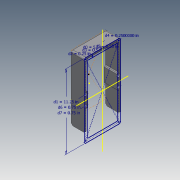
# Autodesk Inventor part: Standard
Saved by Autodesk Inventor 2020.3 (Build 243373000, 373)
## iProperties
RuleStatus: InUse
AfterDocSave0: file://Part Number Cleaner
Created: 2023-01-17
Material: Generic
Catalog Web Link: https://www.janelia.org/
Vendor: HHMI: JRC - jET
Document SubType Name: Modeling
Designer: arnoldj
Density: 1 g/cm^3
Appearance: Default
LAB/DEPT: A. LEE (LAB)
DESIGN DEPARTMENT: HHMI: JRC - jET
ALTERED ITEM PART NUMBER: N/A
ALTERED ITEM VENDOR: N/A
ALTERED ITEM DESCRIPTION: N/A
Title: Standard
Author: arnoldj
Revision Number: 0
Autodesk Inventor part; units mm, degrees
ref_plane "YZ Plane" through (0, 0, 0) normal (1, 0, 0) x (0, 1, 0)
ref_plane "XZ Plane" through (0, 0, 0) normal (0, 1, 0) x (-1, 0, 0)
ref_plane "XY Plane" through (0, 0, 0) normal (0, 0, 1) x (1, 0, 0)
sketch "Sketch1" plane through (0, 0, 0) normal (1, 0, 0) x (0, 1, 0)
  line L0 (0, 99.6312) -> (0, -99.6312) projected
  line L1 (-202.2597, 0) -> (204.2274, 0) projected
  line L2 (-136.525, -69.85) -> (136.525, -69.85)
  line L3 (142.875, -63.5) -> (142.875, 63.5)
  line L4 (136.525, 69.85) -> (-136.525, 69.85)
  line L5 (-142.875, 63.5) -> (-142.875, -63.5)
  line L6 (-142.875, -69.85) -> (142.875, 69.85) construction
  line L7 (142.875, -69.85) -> (-142.875, 69.85) construction
  arc A0 (142.875, 63.5) -> (136.525, 69.85) centre (136.525, 63.5) ccw
  arc A1 (136.525, -69.85) -> (142.875, -63.5) centre (136.525, -63.5) ccw
  arc A2 (-142.875, -63.5) -> (-136.525, -69.85) centre (-136.525, -63.5) ccw
  arc A3 (-136.525, 69.85) -> (-142.875, 63.5) centre (-136.525, 63.5) ccw
  line L8 (130.175, 57.15) -> (130.175, -57.15)
  line L9 (130.175, -57.15) -> (-130.175, -57.15)
  line L10 (-130.175, -57.15) -> (-130.175, 57.15)
  line L11 (-130.175, 57.15) -> (130.175, 57.15)
  line L12 (-136.525, 63.5) -> (136.525, 63.5) construction
  line L13 (136.525, 63.5) -> (136.525, -63.5) construction
  line L14 (136.525, -63.5) -> (-136.525, -63.5) construction
  line L15 (-136.525, -63.5) -> (-136.525, 63.5) construction
  line L16 (-136.525, 63.5) -> (136.525, -63.5) construction
  line L17 (136.525, 63.5) -> (-136.525, -63.5) construction
  point P0 (0, 0)
  point P1 (19.05, 63.5)
  point P2 (19.05, -63.5)
  point P3 (-19.05, 63.5)
  point P4 (-19.05, -63.5)
  dimension "d0" = 139.7
  dimension "d1" = 285.75
  dimension "d2" = 6.35
  dimension "d3" = 12.7
  dimension "d4" = 6.35
  dimension "d5" = 6.35
  dimension "d6" = 19.05
  dimension "d7" = 19.05
  constraints: 32 end point, 12 point on line, 8 point on circle, 8 tangent, 6 parallel, 4 centre point, 4 coincident, 4 midpoint, 3 equal radius, 3 perpendicular, 2 horizontal, 2 vertical alignment, 3 other
  measures "d0" distance of L7.start L6.end
  measures "d1" distance of L6.end L7.end
  measures "d2" radius of A0
  measures "d3" distance between parallel lines of L3 L8
  measures "d4" distance between parallel lines of L14 L2
  measures "d5" distance between parallel lines of L13 L3
  measures "d6" distance from line of L0 point (19.05, 63.5)
  measures "d7" distance from line of point (-19.05, 63.5) L0
extrude "Extrusion1" add sketch "Sketch1" against normal blind 49.53 contours L4 A0 L3 L1 L8 L11 L0 | L0 L11 L10 L1 L5 A3 L4 | L9 L8 L1 L3 A1 L2 L0 | L0 L2 A2 L5 L1 L10 L9
fillet "Fillet1" radius 6.35 4 edges at (-24.765, 130.175, 57.15) (-24.765, 130.175, -57.15) (-24.765, -130.175, -57.15) (-24.765, -130.175, 57.15)
hole "Hole1" at (0, 136.525, 63.5) at (0, 136.525, -63.5) at (0, 19.05, 63.5) at (0, 19.05, -63.5) at (0, -19.05, 63.5) at (0, -19.05, -63.5) at (0, -136.525, 63.5) at (0, -136.525, -63.5) direction (-1, 0, 0) diameter 5.334 end through all counterbore diameter 10.16 counterbore depth 8.89
sketch "Sketch2" plane through (-49.53, 0, 0) normal (-1, 0, 0) x (0, 0, 1)
  line L0 (0, -202.2597) -> (0, 204.2274) projected
  line L1 (99.6312, 0) -> (-99.6312, 0) projected
  line L2 (119.4093, -203.1024) -> (-119.4093, -203.1024)
  line L3 (-119.4093, -203.1024) -> (-119.4093, 0)
  line L4 (-119.4093, 0) -> (119.4093, 0)
  line L5 (119.4093, 0) -> (119.4093, -203.1024)
  line L6 (119.4093, -203.1024) -> (-119.4093, 0) construction
  line L7 (-119.4093, -203.1024) -> (119.4093, 0) construction
  point P0 (0, 0)
  point P1 (0, -101.5512)
  point P2 (119.4093, 0)
  dimension "d18" = 0
  constraints: 12 end point, 2 midpoint, 2 parallel, 1 horizontal, 1 perpendicular, 1 point on line
  measures "d18" distance between parallel lines of L4 L1
extrude "Extrusion2" [suppressed]
sketch "Sketch3" plane through (-34.925, 0, -69.85) normal (0, -1, 0) x (1, 0, 0)
  line L0 (0, 12.7) -> (34.925, 12.7) projected
  line L1 (0, 0) -> (0, 12.7) projected
  line L2 (34.925, 0) -> (0, 0) projected
  line L3 (34.925, 12.7) -> (34.925, 0) projected
  line L4 (34.925, 127) -> (0, 127) projected
  line L5 (34.925, 139.7) -> (34.925, 127) projected
  line L6 (0, 139.7) -> (34.925, 139.7) projected
  line L7 (0, 127) -> (0, 139.7) projected
  line L8 (0, 133.35) -> (0, 6.35) construction
  line L9 (34.925, 6.35) -> (0, 6.35) construction
  line L10 (0, 6.35) -> (34.925, 6.35) construction
  line L11 (0, 133.35) -> (34.925, 133.35) construction
  line L12 (34.925, 135.417) -> (34.925, 131.283) construction
  line L13 (34.925, 133.35) -> (0, 133.35) construction
  point P0 (34.925, 69.85)
  point P1 (7.62, 6.35)
  point P2 (27.305, 6.35)
  point P3 (27.305, 133.35)
  point P4 (7.62, 133.35)
  dimension "d21" = 7.62
  dimension "d22" = 7.62
  dimension "d23" = 7.62
  dimension "d24" = 7.62
  constraints: 4 end point, 4 point on line, 1 collinear, 1 midpoint
  measures "d21" distance from line of L1 point (7.62, 6.35)
  measures "d22" distance from line of point (27.305, 6.35) L3
  measures "d23" distance from line of point (7.62, 133.35) L7
  measures "d24" distance from line of point (27.305, 133.35) L5
hole "Hole2" [suppressed]
chamfer "Chamfer1" [suppressed]
sketch "Sketch4" plane through (-49.53, 0, 0) normal (-1, 0, 0) x (0, 0, 1)
  line L0 (0, -202.2597) -> (0, 204.2274) projected
  line L1 (99.6312, 0) -> (-99.6312, 0) projected
  line L2 (116.354, -104.775) -> (-116.354, -104.775)
  line L3 (-116.354, -104.775) -> (-116.354, -199.2224)
  line L4 (-116.354, -199.2224) -> (116.354, -199.2224)
  line L5 (116.354, -199.2224) -> (116.354, -104.775)
  line L6 (116.354, -104.775) -> (-116.354, -199.2224) construction
  line L7 (-116.354, -104.775) -> (116.354, -199.2224) construction
  line L8 (63.5, 142.875) -> (-63.5, 142.875) projected
  point P0 (0, 0)
  point P1 (0, -151.9987)
  dimension "d35" = 247.65
  constraints: 12 end point, 2 midpoint, 2 parallel, 1 horizontal, 1 perpendicular, 1 point on line
  measures "d35" distance between parallel lines of L2 L8
extrude "Extrusion3" cut sketch "Sketch4" against normal through all
sketch "Sketch5" plane through (-49.53, 0, 0) normal (-1, 0, 0) x (0, 0, 1)
  line L0 (-57.15, -104.775) -> (-57.15, 123.825) projected
  line L1 (-50.8, 130.175) -> (50.8, 130.175) projected
  line L2 (57.15, 123.825) -> (57.15, -104.775) projected
  line L3 (0, -202.2597) -> (0, 204.2274) projected
  arc A0 (-50.8, 130.175) -> (-57.15, 123.825) centre (-50.8, 123.825) ccw projected
  arc A1 (57.15, 123.825) -> (50.8, 130.175) centre (50.8, 123.825) ccw projected
  line L4 (-62.23, -104.775) -> (-62.23, 123.825)
  arc A2 (-50.8, 135.255) -> (-62.23, 123.825) centre (-50.8, 123.825) ccw
  line L5 (-50.8, 135.255) -> (50.8, 135.255)
  arc A3 (62.23, 123.825) -> (50.8, 135.255) centre (50.8, 123.825) ccw
  line L6 (62.23, 123.825) -> (62.23, -104.775)
  line L7 (62.23, -28.575) -> (-62.23, -28.575)
  line L8 (-62.23, -28.575) -> (-62.23, 28.575)
  line L9 (-62.23, 28.575) -> (62.23, 28.575)
  line L10 (62.23, 28.575) -> (62.23, -28.575)
  line L11 (62.23, -28.575) -> (-62.23, 28.575) construction
  line L12 (-62.23, -28.575) -> (62.23, 28.575) construction
  line L13 (-69.85, -104.775) -> (-57.15, -104.775) projected
  line L14 (57.15, -104.775) -> (69.85, -104.775) projected
  point P0 (0, 0)
  point P1 (57.15, 28.575)
  point P2 (-57.15, 28.575)
  point P3 (57.15, -28.575)
  point P4 (-57.15, -28.575)
  dimension "d38" = 5.08
  dimension "d39" = 57.15
  constraints: 18 end point, 4 point on circle, 2 centre point, 2 midpoint, 2 parallel, 1 horizontal, 1 perpendicular, 1 point on line, 4 other
  measures "d38" distance between parallel lines of L1 L5
  measures "d39" distance between parallel lines of L7 L9
extrude "Extrusion4" cut sketch "Sketch5" against normal through all contours L13 L4 L7 L0 | L9 L4 A2 L5 L3 L1 A0 L0 | L7 L6 L14 L2 | L3 L5 A3 L6 L9 L2 A1 L1
fillet "Fillet2" radius 3.175 8 edges at (-24.765, -28.575, -57.15) (-24.765, -28.575, -62.23) (-24.765, 28.575, -57.15) (-24.765, 28.575, -62.23) (-24.765, -28.575, 57.15) (-24.765, -28.575, 62.23) (-24.765, 28.575, 57.15) (-24.765, 28.575, 62.23)
chamfer "Chamfer2" distance 6.35 angle 45 2 edges at (-49.53, -104.775, -66.04) (-49.53, -104.775, 66.04)
sketch "Sketch6" plane through (-49.53, 0, 0) normal (-1, 0, 0) x (0, 0, 1)
  line L0 (69.0599, 146.1578) -> (-63.5, 146.1578) construction
  line L1 (-63.5, 146.1578) -> (-63.5, -84.3884) construction
  line L2 (-63.5, -84.3884) -> (69.0599, -84.3884) construction
  line L3 (69.0599, -84.3884) -> (69.0599, 146.1578) construction
  line L4 (69.0599, 146.1578) -> (-63.5, -84.3884) construction
  line L5 (-63.5, 146.1578) -> (69.0599, -84.3884) construction
  point P0 (0, 0)
  point P1 (2.7799, 30.8847)
  point P2 (63.5, -19.05)
  point P3 (-63.5, 136.525)
  constraints: 12 end point, 2 midpoint, 2 parallel, 1 horizontal, 1 perpendicular, 1 vertical alignment
body "Solid1"
